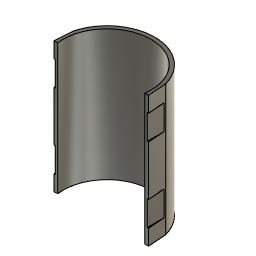
Basic WristStrap For testing (Autodesk Fusion 360 design; units mm, degrees)
Autodesk Fusion 360 part; units mm, degrees
sketch "Sketch1" plane through (0, 0, 0) normal (0, 0, 1) x (1, 0, 0)
  line L0 (0, 0) -> (-70, 0)
  line L1 (-35, 0) -> (-35, 40)
  arc A0 (0, 0) -> (-70, 0) centre (-35, 4.6875) ccw
  line L2 (-70, 0) -> (-73, 0)
  line L3 (0, 0) -> (3, 0)
  line L4 (-35, 40) -> (-35, 43)
  arc A1 (3, 0) -> (-73, 0) centre (-35, 4.7093) ccw
  line L5 (-73, 0) -> (-71.8933, 14.9591)
  line L6 (3, 0) -> (1.8933, 14.9591)
  dimension "d1" = 70
  dimension "d2" = 40
  dimension "d3" = 3
  dimension "d4" = 3
  dimension "d5" = 3
  dimension "d6" = 15
  dimension "d7" = 15
  constraint coincident L0.start A0.start
  constraint horizontal L0
  constraint midpoint L0 L1.start
  constraint perpendicular L0 L1
  constraint coincident L1.end A0
  constraint parallel L0 L2
  constraint parallel L0 L3
  constraint midpoint A0 L1.end
  constraint vertical L4
  constraint coincident L4.end A1
  constraint coincident A1 L5.end
  constraint coincident A1 L6.end
  measures "d1" distance of L0.start L0.end
  measures "d2" distance of L1.start L1.end
  measures "d3" distance of L0.end L2.end
  measures "d4" distance of L0.start L3.end
  measures "d5" distance of L1.end L4.end
  measures "d6" distance of L2.end L5.end
  measures "d7" distance of L3.end L6.end
extrude "Extrude1" add sketch "Sketch1" along normal blind 105 contours A0 L3 L4 A1 L6 | A0 L2 L4 A1 L5
sketch "Sketch4" plane through (0, 0, 0) normal (0, -1, 0) x (1, 0, 0)
  line L0 (-73, 0) -> (-70, 0)
  line L1 (-70, 0) -> (-70, 105)
  line L2 (-70, 105) -> (-73, 105)
  line L3 (-73, 105) -> (-73, 0)
  line L4 (-73, 105) -> (3, 105)
  line L5 (3, 105) -> (3, 0)
  line L6 (3, 0) -> (-73, 0)
  line L7 (-73, 0) -> (-73, 105)
  line L8 (-73, 52.5) -> (-73, 72.5)
  line L9 (-73, 72.5) -> (-73, 92.5)
  line L10 (-73, 92.5) -> (-72, 92.5)
  line L11 (-72, 92.5) -> (-72, 72.5)
  line L12 (-72, 72.5) -> (-73, 72.5)
  line L13 (-73, 72.5) -> (-73, 92.5)
  line L14 (-73, 52.5) -> (3, 52.5) construction
  line L15 (-35, 52.5) -> (-35, 93.5456) construction
  line L16 (-73, 32.5) -> (-73, 12.5)
  line L17 (-72, 12.5) -> (-72, 32.5)
  line L18 (-73, 12.5) -> (-72, 12.5)
  line L19 (-72, 32.5) -> (-73, 32.5)
  line L20 (3, 92.5) -> (2, 92.5)
  line L21 (2, 72.5) -> (3, 72.5)
  line L22 (3, 72.5) -> (3, 92.5)
  line L23 (2, 92.5) -> (2, 72.5)
  line L24 (3, 72.5) -> (3, 92.5)
  line L25 (2, 32.5) -> (3, 32.5)
  line L26 (3, 32.5) -> (3, 12.5)
  line L27 (2, 12.5) -> (2, 32.5)
  line L28 (3, 12.5) -> (2, 12.5)
  dimension "d31" = 20
  dimension "d32" = 20
  dimension "d33" = 1
  dimension "d34" = 76
  constraint horizontal L4
  constraint vertical L5
  constraint horizontal L6
  constraint vertical L7
  constraint coincident L2.end L3.start
  constraint midpoint L7 L8.start
  constraint parallel L7 L8
  constraint parallel L1 L9
  constraint horizontal L10
  constraint vertical L11
  constraint horizontal L12
  constraint vertical L13
  constraint perpendicular L5 L14
  constraint midpoint L14 L15.start
  constraint perpendicular L14 L15
  constraint symmetric L9.end L14 L16.end
  constraint symmetric L10.end L14 L17.start
  constraint symmetric L11.end L14 L17.end
  constraint symmetric L8.end L14 L16.start
  constraint symmetric L8.end L15 L21.end
  constraint symmetric L9.end L15 L20.start
  constraint symmetric L10.end L15 L20.end
  constraint symmetric L11.end L15 L21.start
  constraint symmetric L15 L16.start L25.end
  constraint symmetric L15 L16.end L26.end
  constraint symmetric L15 L17.start L27.start
  constraint symmetric L15 L17.end L25.start
  measures "d31" distance of L8.start L8.end
  measures "d32" distance of L8.end L9.end
  measures "d33" distance of L9.end L10.end
  measures "d34" distance of L8.start L14.end
extrude "Extrude6" cut sketch "Sketch4" against normal blind 20 contours L3 L7 L16 L17 L18 L19 | L5 L25 L26 L27 L28 | L3 L7 L9 L10 L11 L12 L13 | L5 L20 L21 L22 L23 L24
